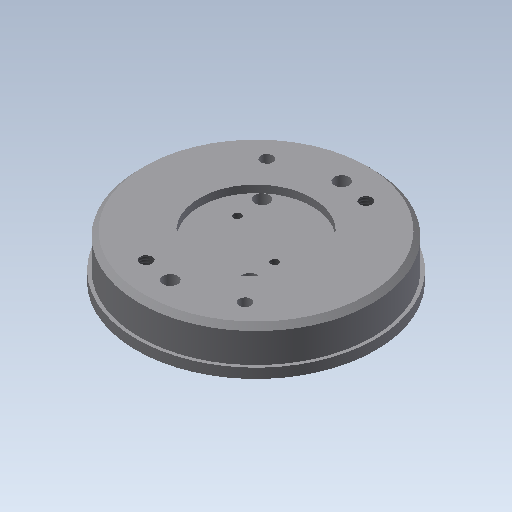
# Autodesk Inventor part: Ledaufnahme
Saved by Autodesk Inventor 2020.2 (Build 242310000, 310)
## iProperties
Part Number: Ledaufnahme
Document SubType Name: Modeling
Density: 1 g/cm^3
Material: Generisch
Appearance: Vorgabe
Mass: 18.2998 g
Surface Area: 56.2692 cm^2
Volume: 18.2998 cm^3
Created: 2020-02-03
Project: 10W LED Lampenkopf
Designer: g.schardt
Control State: 0
Master: False
Checked Out: False
Shininess: 64.0
Length Units: 11269
Angle Units: 11279
Time Units: 11290
Mass Units: 11283
Length Display Precision: 3
Angle Display Precision: 2
Compacted: True
Density: 0.0
Volumn: 0.0
Area: 0.0
PropertySet Name: Model Information
Autodesk Inventor part; units mm, degrees
ref_plane "YZ Plane" through (0, 0, 0) normal (1, 0, 0) x (0, 1, 0)
ref_plane "XZ Plane" through (0, 0, 0) normal (0, 1, 0) x (-1, 0, 0)
ref_plane "XY Plane" through (0, 0, 0) normal (0, 0, 1) x (1, 0, 0)
sketch "Skizze1" plane through (0, 0, 0) normal (0, 0, 1) x (1, 0, 0)
  circle A0 centre (0, 0) radius 24.4
  dimension "d0" = 48.8
  constraints: 1 centre point, 1 coincident
  measures "d0" diameter of A0
extrude "Extrusion1" add sketch "Skizze1" along normal blind 9
sketch "Skizze2" plane through (0, 0, 9) normal (0, 0, 1) x (1, 0, 0)
  circle A0 centre (0, 0) radius 24.4 projected
  circle A1 centre (0, 0) radius 11.5
  dimension "d5" = 23
  constraints: 1 centre point, 1 coincident
  measures "d5" diameter of A1
extrude "Extrusion2" cut sketch "Skizze2" against normal blind 1.5 contours A1
sketch "Skizze10" plane through (0, 0, 9) normal (0, 0, 1) x (1, 0, 0)
  circle A0 centre (0, 0) radius 24.4 projected
  circle A1 centre (0, 0) radius 23.75
  dimension "d62" = 47.5
  constraints: 1 centre point, 1 coincident
  measures "d62" diameter of A1
extrude "Extrusion3" cut sketch "Skizze10" against normal blind 7
sketch "Skizze12" plane through (0, 0, 0) normal (0, 0, -1) x (-1, 0, 0)
  circle A0 centre (0, 0) radius 24.4 projected
  circle A1 centre (0, 0) radius 23.5
  dimension "d82" = 47
  constraints: 1 centre point, 1 coincident
  measures "d82" diameter of A1
extrude "Extrusion4" [suppressed]
sketch "Skizze5" plane through (0, 0, 9) normal (0, 0, 1) x (1, 0, 0)
  circle A0 centre (0, 0) radius 11.5 projected
  circle A1 centre (0, 0) radius 24.4 projected
  circle A2 centre (0, 0) radius 17.5
  point P0 (0, 17.5)
  point P1 (0, -17.5)
  dimension "d17" = 35
  constraints: 2 point on circle, 2 vertical alignment, 1 centre point, 1 coincident
  measures "d17" diameter of A2
hole "Bohrung2" at (0, 17.5, 9) at (0, -17.5, 9) direction (0, 0, -1) diameter 3 end through all
sketch "Skizze6" plane through (0, 0, 9) normal (0, 0, 1) x (1, 0, 0)
  circle A0 centre (0, 17.5) radius 1.5 projected
  circle A1 centre (0, -17.5) radius 1.5 projected
  circle A2 centre (0, 0) radius 11.5 projected
  circle A3 centre (0, 0) radius 24.4 projected
  circle A4 centre (0, 17.5) radius 1.5 projected
  circle A5 centre (0, -17.5) radius 1.5 projected
  circle A6 centre (0, 0) radius 11.5 projected
  circle A7 centre (0, 0) radius 17.5
  point P0 (5.9854, 16.4446)
  point P1 (-5.9854, -16.4446)
  dimension "d25" = 20
  dimension "d26" = 20
  constraints: 3 point on circle, 1 centre point
hole "Bohrung3" at (5.9854, 16.4446, 9) at (-5.9854, -16.4446, 9) direction (0, 0, -1) diameter 2.459 end through all thread size "M3x0.5" class "6H" standard "ANSI Metric M Profile"
sketch "Skizze4" plane through (0, 0, 7.5) normal (0, 0, 1) x (1, 0, 0)
  circle A0 centre (0, 0) radius 11.5 projected
  circle A1 centre (0, 0) radius 6.35
  circle A2 centre (5.9854, 16.4446) radius 1.2295 projected
  circle A3 centre (-5.9854, -16.4446) radius 1.2295 projected
  line L0 (5.9854, 16.4446) -> (-5.9854, -16.4446)
  line L1 (-8.743, 3.1822) -> (10.8065, -3.9332)
  point P0 (5.967, -2.1718)
  point P1 (-5.967, 2.1718)
  dimension "d9" = 12.7
  constraints: 4 end point, 3 point on line, 2 point on circle, 1 centre point, 1 coincident, 1 perpendicular, 2 other
  measures "d9" diameter of A1
hole "Bohrung1" at (5.967, -2.1718, 7.5) at (-5.967, 2.1718, 7.5) direction (0, 0, -1) diameter 1.567 end through all thread size "M2x0.4" class "6H" standard "ISO Metric profile"
chamfer "Fase3" distance 1 angle 45 1 edges at (-23.75, 0, 9)
chamfer "Fase6" [suppressed]
sketch "Skizze15" plane through (0, 0, 9) normal (0, 0, 1) x (1, 0, 0)
  circle A0 centre (0, 0) radius 10 construction
  line L0 (-6.4279, 7.6604) -> (7.0707, -8.4265) construction
  line L1 (0, -34.16) -> (0, 34.16) construction
  line L2 (0, 0) -> (11, 0) construction
  point P0 (6.4279, -7.6604)
  dimension "d110" = 20
  dimension "d111" = 40
  dimension "d115" = 11
  constraints: 4 end point, 2 coincident, 2 point on circle, 2 point on line, 1 centre point, 1 horizontal
  measures "d110" diameter of A0
  measures "d111" angle of L1 L0
  measures "d115" distance of point (0, 0) L0.end
hole "Bohrung9" at (6.4279, -7.6604, 9) at (-6.4279, 7.6604, 9) direction (0, 0, -1) diameter 3 end through all
sketch "Skizze17" plane through (0, 0, 0) normal (0, 0, -1) x (-1, 0, 0)
  circle A0 centre (0, 0) radius 18 construction
  circle A1 centre (0, 0) radius 23.75 construction
  line L0 (11.5702, 13.7888) -> (-11.5702, -13.7888) construction
  point P0 (7.3921, 8.8095)
  point P1 (-7.3921, -8.8095)
  dimension "d134" = 36
  constraints: 3 coincident, 2 end point, 1 centre point
  measures "d134" diameter of A0
hole "Bohrung11" at (11.5702, -13.7888, 0) at (-11.5702, 13.7888, 0) direction (0, 0, 1) diameter 2.459 end through all thread size "M3x0.5" class "6H" standard "ANSI Metric M Profile"
